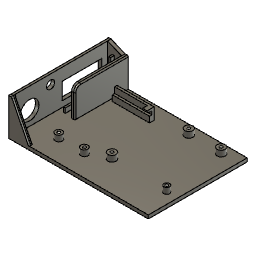
Count Down Case v5 (Autodesk Fusion 360 design; units mm, degrees)
Autodesk Fusion 360 part; units mm, degrees
note: some values were not read from the file. Set by a fixed rule: which sketch regions a step uses.
sketch "Sketch1" plane through (0, 0, 0) normal (0, 1, 0) x (1, 0, 0)
  line L0 (0, 0) -> (120, 0)
  line L1 (120, 0) -> (120, 85)
  line L2 (120, 85) -> (0, 85)
  line L3 (0, 85) -> (0, 0)
  constraint horizontal L0
  constraint vertical L1
  constraint horizontal L2
  constraint vertical L3
  constraint coincident L0.start L3.end
extrude "Extrude1" add sketch "Sketch1" along normal blind 3
sketch "Sketch2" plane through (0, 3, 0) normal (0, 1, 0) x (-1, 0, 0)
  line L0 (0, -85) -> (0, 0)
  line L1 (0, 0) -> (-120, 0)
  line L2 (-120, 0) -> (-120, -85)
  line L3 (-120, -85) -> (0, -85)
  line L4 (-60, -85) -> (-60, 0)
  line L5 (-60, -76.9514) -> (-120, -76.9514)
  line L6 (-77.8086, -80) -> (-77.8086, -73)
  circle A0 centre (-77.8086, -76.9514) radius 3.5
  circle A1 centre (-105.7039, -76.9514) radius 3.5
  dimension "d3" = 7
  dimension "d4" = 7
  constraint midpoint L3 L4.start
  constraint midpoint L1 L4.end
  constraint coincident L4 L5.start
  constraint coincident L2 L5.end
  constraint perpendicular L2 L5
  constraint perpendicular L5 L6
  constraint coincident L5 A0.centre
  constraint coincident L6 A0.centre
  constraint coincident L5 A1.centre
  measures "d3" diameter of A0
  measures "d4" diameter of A1
sketch "Sketch3" plane through (0, 3, 0) normal (0, 1, 0) x (-1, 0, 0)
  line L0 (-60, -10.9513) -> (-119.9962, -10.9513)
  line L1 (-60, -85) -> (-60, 0)
  line L2 (-60, -26.1629) -> (-72, -26.1629)
  line L3 (-62.566, -28.9848) -> (-62.566, -23)
  circle A0 centre (-62.566, -26.1629) radius 3.5
  line L4 (-107.0217, -24.9659) -> (-120.1868, -24.9659)
  line L5 (-110.7456, -28) -> (-110.7456, -22)
  circle A1 centre (-110.7456, -25) radius 2.5
  line L6 (-55, 0) -> (-55.9638, 0)
  line L7 (-55.9638, 0) -> (-55.9638, -85)
  line L8 (-55.9638, -85) -> (-55, -85)
  line L9 (-55, -85) -> (-55, 0)
  line L10 (0, 0) -> (-120, 0)
  line L11 (-120, -85) -> (0, -85)
  dimension "d5" = 7
  dimension "d6" = 5
  constraint horizontal L0
  constraint coincident L1 L2.start
  constraint perpendicular L1 L2
  constraint perpendicular L2 L3
  constraint coincident L2 A0.centre
  constraint coincident L3 A0.centre
  constraint perpendicular L4 L5
  constraint midpoint L5 A1.centre
  constraint horizontal L6
  constraint vertical L7
  constraint horizontal L8
  constraint vertical L9
  constraint coincident L7.end L11
  constraint coincident L6.start L10
  measures "d5" diameter of A0
  measures "d6" diameter of A1
extrude "Extrude2" add sketch "Sketch2" sketch "Sketch3" along normal blind 5 contours L5 A0 | L5 L6 A0 | L5 A1 | L5 A1 | L5 L6 A0 of sketch 2 contours L1 A0 | L1 L2 A0 | L1 L2 A0 | L4 L5 A1 | L4 L5 A1 | L4 L5 A1 | L4 L5 A1
hole "Hole1" at (77.8086, 8, -76.9514) direction (0, -1, 0) diameter 2.529 depth 4 tip angle 180
thread "Thread1" "ISO Metric profile 3.0 M3x0.5 6H"
hole "Hole2" at (105.7039, 8, -76.9514) direction (0, -1, 0) diameter 2.529 depth 4 tip angle 180
thread "Thread2" "ISO Metric profile 3.0 M3x0.5 6H"
hole "Hole3" at (62.566, 8, -26.1629) direction (0, -1, 0) diameter 2.529 depth 4 tip angle 180
thread "Thread3" "ISO Metric profile 3.0 M3x0.5 6H"
hole "Hole4" at (110.7456, 8, -25) direction (0, -1, 0) diameter 2.529 depth 4 tip angle 180
thread "Thread4" "ISO Metric profile 3.0 M3x0.5 6H"
sketch "Sketch4" plane through (0, 3, 0) normal (0, 1, 0) x (-1, 0, 0)
  circle A0 centre (-62.566, -26.1629) radius 3.5
  circle A1 centre (-105.7039, -76.9514) radius 3.5
  circle A2 centre (-77.8086, -76.9514) radius 3.5
  circle A3 centre (-110.7456, -25) radius 2.5
  line L0 (0, -85) -> (0, 0)
  line L1 (0, 0) -> (-120, 0)
  line L2 (-120, 0) -> (-120, -85)
  line L3 (-120, -85) -> (0, -85)
  line L4 (-50, -15) -> (-22, -15)
  line L5 (-22, -15) -> (-22, -70)
  line L6 (-22, -70) -> (-50, -70)
  line L7 (-50, -70) -> (-50, -15)
  line L8 (-22, -18) -> (-50, -18)
  circle A4 centre (-25, -18) radius 3
  circle A5 centre (-47, -18) radius 3
  line L9 (-20, -70) -> (-52, -70)
  line L10 (-52, -70) -> (-52, -69)
  line L11 (-52, -69) -> (-20, -69)
  line L12 (-20, -69) -> (-20, -70)
  dimension "d21" = 6
  dimension "d22" = 6
  constraint horizontal L4
  constraint vertical L5
  constraint horizontal L6
  constraint vertical L7
  constraint coincident L5 L8.start
  constraint coincident L7 L8.end
  constraint perpendicular L7 L8
  constraint coincident L8 A4.centre
  constraint coincident L8 A5.centre
  constraint horizontal L9
  constraint vertical L10
  constraint horizontal L11
  constraint vertical L12
  measures "d21" diameter of A4
  measures "d22" diameter of A5
extrude "Extrude3" add sketch "Sketch4" along normal blind 5 contours L8 A5 | L8 A5 | L8 A4 | L5 L6 L7 L9 L11 | L7 L9 L10 L11 | L8 A4 | L5 L9 L11 L12
hole "Hole5" at (25, 8, -18) direction (0, -1, 0) diameter 2.529 depth 4 tip angle 180
thread "Thread5" "ISO Metric profile 3.0 M3x0.5 6H"
hole "Hole6" at (47, 8, -18) direction (0, -1, 0) diameter 2.529 depth 4 tip angle 180
thread "Thread6" "ISO Metric profile 3.0 M3x0.5 6H"
sketch "Sketch5" plane through (0, 3, 0) normal (0, 1, 0) x (-1, 0, 0)
  circle A0 centre (-47, -18) radius 3
  circle A1 centre (-25, -18) radius 3
  line L0 (-20, -69) -> (-20, -70)
  line L1 (-20, -70) -> (-52, -70)
  line L2 (-52, -70) -> (-52, -69)
  line L3 (-52, -69) -> (-20, -69)
  circle A2 centre (-62.566, -26.1629) radius 3.5
  circle A3 centre (-105.7039, -76.9514) radius 3.5
  circle A4 centre (-77.8086, -76.9514) radius 3.5
  circle A5 centre (-110.7456, -25) radius 2.5
  line L4 (0, -85) -> (0, 0)
  line L5 (0, 0) -> (-120, 0)
  line L6 (-120, 0) -> (-120, -85)
  line L7 (-120, -85) -> (0, -85)
  line L8 (-20, -70) -> (-52, -70)
  line L9 (-52, -70) -> (-52, -73)
  line L10 (-52, -73) -> (-20, -73)
  line L11 (-20, -73) -> (-20, -70)
  constraint horizontal L8
  constraint vertical L9
  constraint horizontal L10
  constraint vertical L11
  constraint coincident L0.end L1.start
extrude "Extrude4" add sketch "Sketch5" along normal blind 5 contours L1 L8 L9 L10 L11
sketch "Sketch6" plane through (0, 8, 0) normal (0, 1, 0) x (-1, 0, 0)
  line L0 (-20, -69) -> (-52, -69)
  line L1 (-52, -69) -> (-52, -73)
  line L2 (-52, -73) -> (-20, -73)
  line L3 (-20, -73) -> (-20, -69)
  line L4 (-20, -73) -> (-52, -73)
  line L5 (-52, -73) -> (-52, -71)
  line L6 (-52, -71) -> (-20, -71)
  line L7 (-20, -71) -> (-20, -73)
  constraint horizontal L4
  constraint vertical L5
  constraint horizontal L6
  constraint vertical L7
  constraint midpoint L1 L5.end
  constraint coincident L2.end L3.start
extrude "Extrude5" add sketch "Sketch6" along normal blind 5 contours L1 L2 L3 L4 L5 L6 L7
sketch "Sketch7" plane through (0, 0, -71) normal (0, 0, 1) x (1, 0, 0)
  line L0 (20, 8) -> (52, 8)
  line L1 (52, 8) -> (52, 13)
  line L2 (52, 13) -> (20, 13)
  line L3 (20, 13) -> (20, 8)
  line L4 (48.0761, 13) -> (52, 13)
  line L5 (52, 13) -> (52, 10.5)
  line L6 (52, 10.5) -> (48.0761, 10.5)
  line L7 (48.0761, 10.5) -> (48.0761, 13)
  constraint horizontal L4
  constraint vertical L5
  constraint horizontal L6
  constraint vertical L7
  constraint midpoint L1 L5.end
  constraint coincident L2 L4.start
extrude "Extrude6" add sketch "Sketch7" along normal blind 4 contours L1 L2 L4 L5 L6 L7
sketch "Sketch8" plane through (52, 0, 0) normal (1, 0, 0) x (0, 0, -1)
  line L0 (69, 3) -> (73, 3)
  line L1 (73, 3) -> (73, 13)
  line L2 (73, 13) -> (67, 13)
  line L3 (67, 13) -> (67, 10.5)
  line L4 (67, 10.5) -> (71, 10.5)
  line L5 (71, 10.5) -> (71, 8)
  line L6 (71, 8) -> (69, 8)
  line L7 (69, 8) -> (69, 3)
  line L8 (67, 11.75) -> (71, 10.5)
  constraint midpoint L3 L8.start
  constraint coincident L4.end L5.start
extrude "Extrude7" cut sketch "Sketch8" against normal blind 4 contours L3 L4 L8
sketch "Sketch9" plane through (0, 3, 0) normal (0, 1, 0) x (-1, 0, 0)
  line L0 (-52, -73) -> (-52, -69)
  line L1 (-52, -69) -> (-20, -69)
  line L2 (-20, -69) -> (-20, -73)
  line L3 (-20, -73) -> (-52, -73)
  circle A0 centre (-47, -18) radius 3
  circle A1 centre (-25, -18) radius 3
  circle A2 centre (-62.566, -26.1629) radius 3.5
  circle A3 centre (-105.7039, -76.9514) radius 3.5
  circle A4 centre (-77.8086, -76.9514) radius 3.5
  circle A5 centre (-110.7456, -25) radius 2.5
  line L4 (0, -85) -> (0, 0)
  line L5 (0, 0) -> (-120, 0)
  line L6 (-120, 0) -> (-120, -85)
  line L7 (-120, -85) -> (0, -85)
  line L8 (0, 0) -> (-2.9371, 0)
  line L9 (-2.9371, 0) -> (-2.9371, -85)
  line L10 (-2.9371, -85) -> (0, -85)
  line L11 (0, -85) -> (0, 0)
  line L12 (0, 0) -> (-3, 0)
  line L13 (-3, 0) -> (-3, -85)
  line L14 (-3, -85) -> (0, -85)
  line L15 (0, -85) -> (0, 0)
  dimension "d39" = 3
  constraint horizontal L8
  constraint vertical L9
  constraint horizontal L10
  constraint vertical L11
  constraint coincident L7 L9.end
  constraint coincident L4.end L5.start
  constraint horizontal L12
  constraint vertical L13
  constraint horizontal L14
  constraint vertical L15
  constraint coincident L7 L13.end
  measures "d39" distance of L4.end L12.end
extrude "Extrude8" add sketch "Sketch9" along normal blind 30 contours L4 L5 L7 L8 L9 L10 L11 L12 L14 L15
sketch "Sketch10" plane through (2.9371, 0, 0) normal (1, 0, 0) x (0, 0, -1)
  line L0 (0, 3) -> (85, 3)
  line L1 (85, 3) -> (85, 33)
  line L2 (85, 33) -> (0, 33)
  line L3 (0, 33) -> (0, 3)
  line L4 (0, 33) -> (3, 33)
  line L5 (3, 33) -> (3, 3)
  line L6 (3, 3) -> (0, 3)
  line L7 (0, 3) -> (0, 33)
  line L8 (85, 33) -> (82, 33)
  line L9 (82, 33) -> (82, 3)
  line L10 (82, 3) -> (85, 3)
  line L11 (85, 3) -> (85, 33)
  dimension "d42" = 3
  dimension "d43" = 3
  constraint horizontal L4
  constraint vertical L5
  constraint horizontal L6
  constraint vertical L7
  constraint coincident L0 L5.end
  constraint coincident L2.end L3.start
  constraint horizontal L8
  constraint vertical L9
  constraint horizontal L10
  constraint vertical L11
  constraint coincident L0 L9.end
  constraint coincident L1.end L2.start
  measures "d42" distance of L2.end L4.end
  measures "d43" distance of L1.end L8.end
extrude "Extrude9" add sketch "Sketch10" along normal blind 15 contours L0 L2 L3 L4 L5 L6 L7 | L0 L1 L2 L8 L9 L10 L11
sketch "Sketch11" plane through (0, 0, -3) normal (0, 0, -1) x (-1, 0, 0)
  line L0 (-2.9371, 3) -> (-2.9371, 33)
  line L1 (-2.9371, 33) -> (-17.9371, 33)
  line L2 (-17.9371, 33) -> (-17.9371, 3)
  line L3 (-17.9371, 3) -> (-2.9371, 3)
  line L4 (-2.9371, 33) -> (-17.9371, 3)
  constraint coincident L0.end L1.start
  constraint coincident L2.end L3.start
extrude "Extrude10" cut sketch "Sketch11" against normal blind 4 contours L1 L2 L4
sketch "Sketch13" plane through (0, 3, 0) normal (0, 1, 0) x (-1, 0, 0)
  line L0 (-17.9371, -82) -> (-2.9371, -82)
  line L1 (-2.9371, -82) -> (-2.9371, -3)
  line L2 (-2.9371, -3) -> (-17.9371, -3)
  line L3 (-17.9371, -3) -> (-17.9371, 0)
  line L4 (-17.9371, 0) -> (-120, 0)
  line L5 (-120, 0) -> (-120, -85)
  line L6 (-120, -85) -> (-17.9371, -85)
  line L7 (-52, -73) -> (-52, -69)
  line L8 (-52, -69) -> (-20, -69)
  line L9 (-20, -69) -> (-20, -73)
  line L10 (-20, -73) -> (-52, -73)
  circle A0 centre (-47, -18) radius 3
  circle A1 centre (-25, -18) radius 3
  circle A2 centre (-62.566, -26.1629) radius 3.5
  circle A3 centre (-105.7039, -76.9514) radius 3.5
  circle A4 centre (-77.8086, -76.9514) radius 3.5
  circle A5 centre (-110.7456, -25) radius 2.5
  line L11 (-14.9586, -82) -> (-17.7256, -82)
  line L12 (-17.7256, -82) -> (-17.7256, -39)
  line L13 (-17.7256, -39) -> (-14.9586, -39)
  line L14 (-14.9586, -39) -> (-14.9586, -82)
  line L15 (-17.9371, -85) -> (-17.9371, -82)
  constraint horizontal L11
  constraint vertical L12
  constraint horizontal L13
  constraint vertical L14
  constraint coincident L0 L11.start
extrude "Extrude12" add sketch "Sketch13" along normal blind 25 contours L0 L11 L12 L13 L14
sketch "Sketch14" plane through (0, 0, -82) normal (0, 0, 1) x (1, 0, 0)
  line L0 (17.7256, 28) -> (17.7256, 3)
  line L1 (17.7256, 3) -> (17.9371, 3)
  line L2 (17.9371, 3) -> (17.9371, 33)
  line L3 (17.9371, 33) -> (2.9371, 33)
  line L4 (2.9371, 33) -> (2.9371, 3)
  line L5 (2.9371, 3) -> (14.9586, 3)
  line L6 (14.9586, 3) -> (14.9586, 28)
  line L7 (14.9586, 28) -> (17.7256, 28)
  line L8 (2.9371, 33) -> (14.9586, 28)
  constraint coincident L3.end L4.start
  constraint coincident L6.end L7.start
extrude "Extrude13" cut sketch "Sketch14" against normal blind 4 contours L0 L1 L2 L3 L7 L8
sketch "Sketch15" plane through (0, 0, 0) normal (-1, 0, 0) x (0, 0, 1)
  line L0 (-85, 0) -> (0, 0)
  line L1 (0, 0) -> (0, 33)
  line L2 (0, 33) -> (-85, 33)
  line L3 (-85, 33) -> (-85, 0)
  line L4 (-77, 8) -> (-43, 8)
  line L5 (-43, 8) -> (-43, 22.5)
  line L6 (-43, 22.5) -> (-77, 22.5)
  line L7 (-77, 22.5) -> (-77, 8)
  dimension "d54" = 34
  dimension "d55" = 14.5
  constraint horizontal L4
  constraint vertical L5
  constraint horizontal L6
  constraint vertical L7
  measures "d54" distance of L4.start L4.end
  measures "d55" distance of L4.start L6.end
extrude "Extrude14" cut sketch "Sketch15" against normal blind 5 contours L4 L5 L6 L7
sketch "Sketch16" plane through (0, 0, 0) normal (-1, 0, 0) x (0, 0, 1)
  line L0 (-43, 8) -> (-77, 8)
  line L1 (-77, 8) -> (-77, 22.5)
  line L2 (-77, 22.5) -> (-43, 22.5)
  line L3 (-43, 22.5) -> (-43, 8)
  line L4 (-85, 0) -> (0, 0)
  line L5 (0, 0) -> (0, 33)
  line L6 (0, 33) -> (-85, 33)
  line L7 (-85, 33) -> (-85, 0)
  circle A0 centre (-15, 15) radius 8
  circle A1 centre (-33, 25) radius 3.5
  dimension "d58" = 16
  dimension "d59" = 7
  measures "d58" diameter of A0
  measures "d59" diameter of A1
extrude "Extrude15" cut sketch "Sketch16" against normal blind 4 contours A0 | A1
fillet "Fillet1" radius 5 1 edges at (16.3421, 28, -39)
fillet "Fillet2" radius 1 4 edges at (1.4685, 33, 0) (10.4371, 18, 0) (10.4371, 18, -3) (0, 33, -42.5)
fillet "Fillet3" radius 1 3 edges at (17.7256, 13, -39) (17.7256, 26.5355, -40.4645) (17.7256, 28, -64.5)
sketch "Sketch17" plane through (0, 3, 0) normal (0, 1, 0) x (-1, 0, 0)
  circle A0 centre (-110.7456, -25) radius 2.5
  circle A1 centre (-77.8086, -76.9514) radius 3.5
  circle A2 centre (-105.7039, -76.9514) radius 3.5
  circle A3 centre (-62.566, -26.1629) radius 3.5
  circle A4 centre (-25, -18) radius 3
  circle A5 centre (-47, -18) radius 3
  line L0 (-52, -73) -> (-52, -69)
  line L1 (-52, -69) -> (-20, -69)
  line L2 (-20, -69) -> (-20, -73)
  line L3 (-20, -73) -> (-52, -73)
  line L4 (-16.7256, -39) -> (-14.9586, -39)
  line L5 (-14.9586, -39) -> (-14.9586, -82)
  line L6 (-14.9586, -82) -> (-2.9371, -82)
  line L7 (-2.9371, -82) -> (-2.9371, -3)
  line L8 (-2.9371, -3) -> (-16.8191, -3)
  ellipse E0 centre (-16.8191, -2) end of major axis (-17.9371, -2) minor radius 1 (-17.9371, -2) -> (-16.8191, -3) ccw
  line L9 (-17.9371, -2) -> (-17.9371, -1)
  ellipse E1 centre (-16.8191, -1) end of major axis (-17.9371, -1) minor radius 1 (-16.8191, 0) -> (-17.9371, -1) ccw
  line L10 (-16.8191, 0) -> (-120, 0)
  line L11 (-120, 0) -> (-120, -85)
  line L12 (-120, -85) -> (-17.7256, -85)
  line L13 (-17.7256, -85) -> (-17.7256, -40)
  arc A6 (-16.7256, -39) -> (-17.7256, -40) centre (-16.7256, -40) ccw
  line L14 (-8.6438, -82) -> (-7, -82)
  line L15 (-7, -82) -> (-7, -40)
  line L16 (-7, -40) -> (-8.6438, -40)
  line L17 (-8.6438, -40) -> (-8.6438, -82)
  constraint horizontal L14
  constraint vertical L15
  constraint horizontal L16
  constraint vertical L17
  constraint coincident L6 L14.start
extrude "Extrude16" add sketch "Sketch17" along normal blind 4 contours L6 L14 L15 L16 L17
sketch "Sketch18" plane through (0, 0, -82) normal (0, 0, 1) x (1, 0, 0)
  line L0 (8.6438, 7) -> (8.6438, 3)
  line L1 (8.6438, 3) -> (14.9586, 3)
  line L2 (14.9586, 3) -> (14.9586, 28)
  line L3 (14.9586, 28) -> (2.9371, 33)
  line L4 (2.9371, 33) -> (2.9371, 3)
  line L5 (2.9371, 3) -> (7, 3)
  line L6 (7, 3) -> (7, 7)
  line L7 (7, 7) -> (8.6438, 7)
  line L8 (7, 7) -> (8.6319, 7)
  line L9 (8.6319, 7) -> (8.6319, 25.0515)
  line L10 (8.6319, 25.0515) -> (7, 25.0515)
  line L11 (7, 25.0515) -> (7, 7)
  constraint horizontal L8
  constraint vertical L9
  constraint horizontal L10
  constraint vertical L11
  constraint coincident L6.end L7.start
extrude "Extrude17" add sketch "Sketch18" along normal blind 3 contours L7 L8 L9 L10 L11
